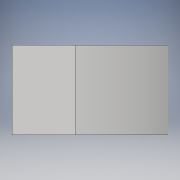
# Autodesk Inventor part: air_skidpad
Saved by Autodesk Inventor 2018.2 (Build 222227000, 227)
## iProperties
Created: 2018-03-06
Part Number: air_skidpad
Material: 一般
Document SubType Name: Modeling
Designer: ku_sk
Density: 1 g/cm^3
Appearance: 既定
Author: ku_sk
Autodesk Inventor part; units mm, degrees
ref_plane "YZ Plane" through (0, 0, 0) normal (1, 0, 0) x (0, 1, 0)
ref_plane "XZ Plane" through (0, 0, 0) normal (0, 1, 0) x (-1, 0, 0)
ref_plane "XY Plane" through (0, 0, 0) normal (0, 0, 1) x (1, 0, 0)
sketch "スケッチ1" plane through (0, 0, 0) normal (0, 0, 1) x (1, 0, 0)
  arc A0 (7513.0096, -1611.9904) -> (-7513.0096, -1611.9904) centre (0, -9125) ccw
  arc A1 (5391.6892, -3733.3108) -> (-5391.6892, -3733.3108) centre (0, -9125) ccw
  line L0 (0, -11250) -> (0, 3625) projected
  line L1 (0, 1500) -> (0, -1500)
  line L2 (-7513.0096, -1611.9904) -> (-5391.6892, -3733.3108)
  line L3 (7513.0096, -1611.9904) -> (5391.6892, -3733.3108)
  point P0 (0, 0)
  dimension "d0" = 3000
  dimension "d1" = 7625
  dimension "d2" = 90
  constraints: 6 end point, 6 point on circle, 4 line through centre, 2 centre point, 2 point on line, 1 collinear, 1 concentric, 1 midpoint
  measures "d0" radial gap between concentric circles of A1 A0
  measures "d1" radius of A1
  measures "d2" angle of L3 L2
extrude "押し出し1" add sketch "スケッチ1" along normal blind 2893.556 and the other way blind 106.444
